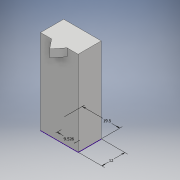
# Autodesk Inventor part: dialPointer
Saved by Autodesk Inventor 2018 (Build 220112000, 112)
## iProperties
Created: 2018-03-03
Part Number: dialPointer
Material: Generic
Document SubType Name: Modeling
Designer: Prakash
Density: 1 g/cm^3
Appearance: Default
Author: Prakash
Autodesk Inventor part; units mm, degrees
ref_plane "YZ Plane" through (0, 0, 0) normal (1, 0, 0) x (0, 1, 0)
ref_plane "XZ Plane" through (0, 0, 0) normal (0, 1, 0) x (-1, 0, 0)
ref_plane "XY Plane" through (0, 0, 0) normal (0, 0, 1) x (1, 0, 0)
sketch "Sketch1" plane through (0, 0, 0) normal (0, 0, 1) x (1, 0, 0)
  line L0 (0, 0) -> (19.5, 0)
  line L1 (19.5, 0) -> (19.5, 12)
  line L2 (19.5, 12) -> (0, 12)
  line L3 (0, 12) -> (0, 0)
  line L4 (4.987, 6) -> (14.513, 6) construction
  line L5 (14.513, 6) -> (19.5, 6)
  line L6 (4.987, 6) -> (0, 6)
  point P0 (0, 6)
  dimension "d0" = 19.5
  dimension "d1" = 12
  dimension "d2" = 9.526
  constraints: 14 end point, 3 midpoint, 3 perpendicular, 2 horizontal, 2 parallel, 1 collinear, 1 point on line
  measures "d0" distance of L1.end L2.end
  measures "d1" distance of L0.end L1.end
  measures "d2" distance of L4.end L4.start
extrude "Extrusion1" add sketch "Sketch1" along normal blind 44
sketch "Sketch3" plane through (0, 0, 44) normal (0, 0, 1) x (1, 0, 0)
  line L0 (0, 0) -> (19.5, 0) projected
  line L1 (5.75, 0) -> (9.75, -5)
  line L2 (9.75, -5) -> (13.75, 0)
  line L3 (9.75, 0) -> (9.75, -5)
  dimension "d6" = 4
  dimension "d7" = 4
  dimension "d8" = 5
  constraints: 6 end point, 2 point on line, 1 midpoint, 1 vertical
  measures "d6" distance of L1.start L3.start
  measures "d7" distance of L2.end L3.start
  measures "d8" vertical distance of L1.end L2.end
extrude "Extrusion2" add sketch "Sketch3" against normal blind 4
equation "\"d7\" = d6"
body "Solid1"
